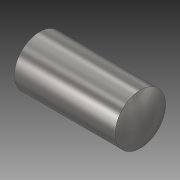
# Autodesk Inventor part: DIN 7 - 3 m6 x 6
Saved by Autodesk Inventor 2019.4 (Build 234330000, 330)
## iProperties
Part Number: DIN 7 - 3 m6 x 6
Material: Edelstahl, austenitisch
Document SubType Name: Modeling
Designer: rYan
Mass: 0.365502 g
Surface Area: 0.719582 cm^2
Volume: 0.0456878 cm^3
Density: 8 g/cm^3
Appearance: Halbpoliert
Author: rYan
Autodesk Inventor part; units mm, degrees
ref_plane "YZ Plane" through (0, 0, 0) normal (1, 0, 0) x (0, 1, 0)
ref_plane "XZ Plane" through (0, 0, 0) normal (0, 1, 0) x (-1, 0, 0)
ref_plane "XY Plane" through (0, 0, 0) normal (0, 0, 1) x (1, 0, 0)
sketch "Skizze1" plane through (0, 0, 0) normal (0, 0, 1) x (1, 0, 0)
  line L0 (3, 1.5) -> (-3, 1.5)
  arc A0 (-3, 1.5) -> (-3.45, 0) centre (-0.725, 0) ccw
  arc A1 (3.45, 0) -> (3, 1.5) centre (0.725, 0) ccw
  line L1 (0, 1.8396) -> (0, -0.3066) projected
  line L2 (-3.45, 0) -> (3.45, 0)
  point P0 (0, 0)
  point P1 (-0.2744, 0)
  dimension "d0" = 6
  dimension "d3" = 3
  dimension "d4" = 0.45
  constraints: 4 end point, 4 point on circle, 2 centre point, 2 horizontal, 2 point on line, 1 midpoint, 1 other
  measures "d0" distance of L0.end L0.start
  measures "d3" diameter of L0 L2
  measures "d4" horizontal distance of L0.start L2.end
revolve "Umdrehung1" add sketch "Skizze1" angle 360 about axis through (-3.45, 0, 0) along (1, 0, 0)
